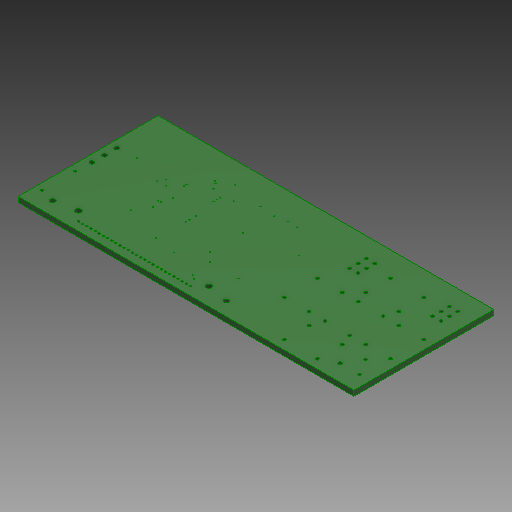
# Autodesk Inventor part: Display.brd_Kontur
Saved by Autodesk Inventor 2017.3 (Build 213256000, 256)
## iProperties
Part Number: Display.brd_Kontur
Material: Generisch
Document SubType Name: Modeling
Designer: Nils
Density: 1 g/cm^3
Appearance: Board-Kontur
Author: Nils
Autodesk Inventor part; units mm, degrees
ref_plane "YZ Plane" through (0, 0, 0) normal (1, 0, 0) x (0, 1, 0)
ref_plane "XZ Plane" through (0, 0, 0) normal (0, 1, 0) x (-1, 0, 0)
ref_plane "XY Plane" through (0, 0, 0) normal (0, 0, 1) x (1, 0, 0)
sketch "Skizze1" plane through (0, 0, 0) normal (0, 0, 1) x (1, 0, 0)
  line L0 (-3.81, 0) -> (99.04, 0)
  line L1 (99.04, 0) -> (99.04, 42.85)
  line L2 (99.04, 42.85) -> (-3.81, 42.85)
  line L3 (-3.81, 42.85) -> (-3.81, 0)
  circle A0 centre (-1.52, 27.94) radius 0.66
  circle A1 centre (93.98, 36.83) radius 0.455
  circle A2 centre (91.44, 36.83) radius 0.455
  circle A3 centre (93.98, 34.29) radius 0.455
  circle A4 centre (91.44, 34.29) radius 0.455
  circle A5 centre (93.98, 31.75) radius 0.455
  circle A6 centre (91.44, 31.75) radius 0.455
  circle A7 centre (68.58, 36.83) radius 0.455
  circle A8 centre (66.04, 36.83) radius 0.455
  circle A9 centre (68.58, 34.29) radius 0.455
  circle A10 centre (66.04, 34.29) radius 0.455
  circle A11 centre (68.58, 31.75) radius 0.455
  circle A12 centre (66.04, 31.75) radius 0.455
  circle A13 centre (95.71, 5.08) radius 0.4
  circle A14 centre (92.71, 9.88) radius 0.4
  circle A15 centre (89.71, 5.08) radius 0.5
  circle A16 centre (-1.78, 15.49) radius 0.405
  circle A17 centre (-1.78, 5.33) radius 0.405
  circle A18 centre (-1.52, 24.13) radius 0.66
  circle A19 centre (76.2, 24.13) radius 0.455
  circle A20 centre (76.2, 13.97) radius 0.455
  circle A21 centre (83.82, 24.13) radius 0.455
  circle A22 centre (83.82, 13.97) radius 0.455
  circle A23 centre (63.7, 24.13) radius 0.455
  circle A24 centre (63.7, 13.97) radius 0.455
  circle A25 centre (71.32, 24.13) radius 0.455
  circle A26 centre (71.32, 13.97) radius 0.455
  circle A27 centre (88.7, 24.13) radius 0.455
  circle A28 centre (88.7, 13.97) radius 0.455
  circle A29 centre (96.32, 24.13) radius 0.455
  circle A30 centre (96.32, 13.97) radius 0.455
  circle A31 centre (85.09, 35.36) radius 0.455
  circle A32 centre (74.93, 35.36) radius 0.455
  circle A33 centre (85.09, 27.74) radius 0.455
  circle A34 centre (74.93, 27.74) radius 0.455
  circle A35 centre (85.09, 10.36) radius 0.455
  circle A36 centre (74.93, 10.36) radius 0.455
  circle A37 centre (85.09, 2.74) radius 0.455
  circle A38 centre (74.93, 2.74) radius 0.455
  circle A39 centre (-1.52, 20.32) radius 0.66
  circle A40 centre (41.27, 2.61) radius 0.3
  circle A41 centre (45.09, 2.61) radius 0.3
  circle A42 centre (42.55, 2.61) radius 0.3
  circle A43 centre (9.21, 5.41) radius 0.85
  circle A44 centre (43.82, 2.61) radius 0.3
  circle A45 centre (13.34, 2.61) radius 0.3
  circle A46 centre (23.5, 2.61) radius 0.3
  circle A47 centre (24.77, 2.61) radius 0.3
  circle A48 centre (22.23, 2.61) radius 0.3
  circle A49 centre (20.96, 2.61) radius 0.3
  circle A50 centre (26.04, 2.61) radius 0.3
  circle A51 centre (46.36, 2.61) radius 0.3
  circle A52 centre (40.01, 2.61) radius 0.3
  circle A53 centre (38.73, 2.61) radius 0.3
  circle A54 centre (37.47, 2.61) radius 0.3
  circle A55 centre (36.2, 2.61) radius 0.3
  circle A56 centre (34.93, 2.61) radius 0.3
  circle A57 centre (33.66, 2.61) radius 0.3
  circle A58 centre (32.38, 2.61) radius 0.3
  circle A59 centre (31.12, 2.61) radius 0.3
  circle A60 centre (49.21, 5.41) radius 0.85
  circle A61 centre (12.07, 2.61) radius 0.3
  circle A62 centre (14.61, 2.61) radius 0.3
  circle A63 centre (15.88, 2.61) radius 0.3
  circle A64 centre (17.14, 2.61) radius 0.3
  circle A65 centre (18.41, 2.61) radius 0.3
  circle A66 centre (19.69, 2.61) radius 0.3
  circle A67 centre (29.85, 2.61) radius 0.3
  circle A68 centre (27.3, 2.61) radius 0.3
  circle A69 centre (28.58, 2.61) radius 0.3
  circle A70 centre (2.61, 4.16) radius 0.75
  circle A71 centre (55.81, 4.16) radius 0.75
  circle A72 centre (24.003, 32.004) radius 0.175
  circle A73 centre (34.925, 9.017) radius 0.175
  circle A74 centre (16.002, 25.527) radius 0.175
  circle A75 centre (14.351, 27.178) radius 0.175
  circle A76 centre (40.64, 34.036) radius 0.175
  circle A77 centre (26.416, 36.322) radius 0.175
  circle A78 centre (4.191, 28.448) radius 0.175
  circle A79 centre (43.815, 5.842) radius 0.175
  circle A80 centre (28.321, 10.033) radius 0.175
  circle A81 centre (17.145, 13.589) radius 0.175
  circle A82 centre (40.259, 24.765) radius 0.175
  circle A83 centre (40.259, 14.605) radius 0.175
  circle A84 centre (51.689, 11.938) radius 0.175
  circle A85 centre (30.48, 31.75) radius 0.175
  circle A86 centre (47.117, 34.544) radius 0.175
  circle A87 centre (44.196, 34.671) radius 0.175
  circle A88 centre (35.941, 34.417) radius 0.175
  circle A89 centre (13.4541, 25.2809) radius 0.175
  circle A90 centre (42.926, 11.938) radius 0.175
  circle A91 centre (22.225, 34.29) radius 0.175
  circle A92 centre (18.796, 20.32) radius 0.175
  circle A93 centre (22.987, 33.655) radius 0.175
  circle A94 centre (19.558, 20.32) radius 0.175
  circle A95 centre (19.558, 17.907) radius 0.175
  circle A96 centre (45.085, 5.08) radius 0.175
  circle A97 centre (18.796, 28.956) radius 0.175
  circle A98 centre (27.432, 30.607) radius 0.175
  circle A99 centre (27.432, 29.591) radius 0.175
  circle A100 centre (27.432, 28.575) radius 0.175
  circle A101 centre (54.864, 27.305) radius 0.175
  circle A102 centre (28.575, 22.098) radius 0.175
  circle A103 centre (28.575, 20.066) radius 0.175
  circle A104 centre (28.575, 18.923) radius 0.175
  circle A105 centre (20.32, 23.241) radius 0.175
  circle A106 centre (18.796, 28.194) radius 0.175
  constraints: 107 centre point, 8 end point
extrude "Display.brd_Kontur" add sketch "Skizze1" along normal blind 1.6
